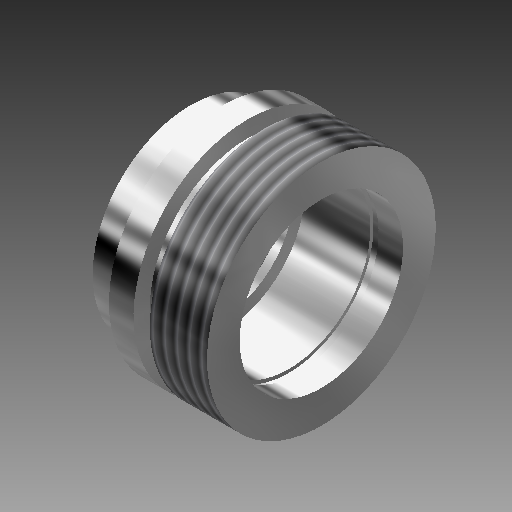
# Autodesk Inventor part: 405-02
Saved by Autodesk Inventor 2019 (Build 230136000, 136)
## iProperties
Company: Autodesk Inc.
Created: 2017-06-27
Part Number: 405-02
Material: Steel, Mild
Document SubType Name: Modeling
Designer: Autodesk Inc.
Mass: 3.82666 g
Surface Area: 8.43889 cm^2
Volume: 0.487473 cm^3
Density: 7.85 g/cm^3
Appearance: Chrome - Polished
Author: Inventor
Autodesk Inventor part; units mm, degrees
ref_plane "YZ Plane" through (0, 0, 0) normal (1, 0, 0) x (0, 1, 0)
ref_plane "XZ Plane" through (0, 0, 0) normal (0, 1, 0) x (-1, 0, 0)
ref_plane "XY Plane" through (0, 0, 0) normal (0, 0, 1) x (1, 0, 0)
sketch "Sketch1" plane through (0, 0, 0) normal (0, 0, 1) x (1, 0, 0)
  line L0 (0, 4.25) -> (2, 4.25)
  line L1 (2, 4.25) -> (2, 6)
  line L2 (2, 6) -> (0, 6)
  line L3 (0, 6) -> (0, 4.25)
  line L4 (2, 5) -> (8, 5)
  line L5 (8, 5) -> (8, 7)
  line L6 (8, 7) -> (2, 7)
  line L7 (2, 7) -> (2, 5)
  line L8 (0, 0) -> (3.6589, 0)
  line L9 (3.5, 7) -> (4.5, 7)
  line L10 (4.5, 7) -> (4.5, 6)
  line L11 (4.5, 6) -> (3.5, 6)
  line L12 (3.5, 6) -> (3.5, 7)
  line L13 (6.5, 5) -> (6, 5)
  line L14 (6, 5) -> (6, 5.2)
  line L15 (6, 5.2) -> (6.5, 5.2)
  line L16 (6.5, 5.2) -> (6.5, 5)
  dimension "d0" = 8.5
  dimension "d1" = 14
  dimension "d2" = 12
  dimension "d3" = 10
  dimension "d4" = 8
  dimension "d5" = 2
  dimension "d6" = 3.5
  dimension "d7" = 4.5
  dimension "d8" = 1
  dimension "d15" = 0.5
  dimension "d16" = 0.2
  dimension "d17" = 1.5
  constraints: 34 end point, 8 parallel, 5 perpendicular, 4 horizontal, 4 point on line, 1 coincident
  measures "d0" diameter of L0 L8
  measures "d1" diameter of L6 L8
  measures "d2" diameter of L2 L8
  measures "d3" diameter of L4 L8
  measures "d4" distance between parallel lines of L5 L3
  measures "d5" distance of L1.end L2.end
  measures "d6" distance between parallel lines of L12 L3
  measures "d7" distance between parallel lines of L10 L3
  measures "d8" distance between parallel lines of L11 L4
  measures "d15" distance of L14.end L15.end
  measures "d16" distance of L13.end L14.end
  measures "d17" distance between parallel lines of L5 L16
revolve "Revolution1" add sketch "Sketch1" angle 360 about axis through (0, 0, 0) along (1, 0, 0) contours L3 L2 L1 L0 | L1 L7 L6 L12 L11 L10 L5 L4 L16 L15 L14
thread "Thread1" size "M14x0.75" class "6g" standard "ANSI Metric M Profile" full length
chamfer "Chamfer1" distance 1.5 angle 45 1 edges at (0, -4.25, 0)
body "Solid1"
